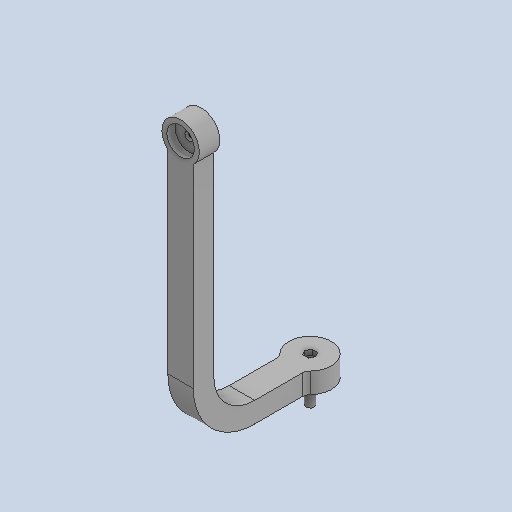
# Autodesk Inventor part: distal_link_2
Saved by Autodesk Inventor 2024 (Build 280153000, 153)
## iProperties
Created: 2023-10-30
Part Number: distal_link_2
Material: Generic
Document SubType Name: Modeling
Designer: MATEO
Density: 1 g/cm^3
Appearance: Default
Author: MATEO
Autodesk Inventor part; units mm, degrees
ref_plane "YZ Plane" through (0, 0, 0) normal (1, 0, 0) x (0, 1, 0)
ref_plane "XZ Plane" through (0, 0, 0) normal (0, 1, 0) x (-1, 0, 0)
sketch "Sketch1" plane through (0, 0, 0) normal (0, 1, 0) x (-1, 0, 0)
  arc A0 (-8.9286, 8.7482) -> (8.9286, 8.7482) centre (0, 0) ccw
  line L0 (-7.5, 12.2474) -> (-7.5, 20)
  line L1 (7.5, 20) -> (7.5, 12.2474)
  line L2 (7.5, 20) -> (-7.5, 20)
  arc A1 (7.5, 12.2474) -> (8.9286, 8.7482) centre (12.5, 12.2474) ccw
  arc A2 (-8.9286, 8.7482) -> (-7.5, 12.2474) centre (-12.5, 12.2474) ccw
  point P0 (7.5, 10)
  point P1 (-7.5, 10)
  point P2 (0, 10)
  point P3 (0, 20)
  dimension "d0" = 25
  dimension "d109" = 5
  dimension "d129" = 15
  dimension "d131" = 10
  constraints: 8 point on circle, 6 end point, 5 horizontal alignment, 4 tangent, 3 centre point, 2 point on line, 2 vertical alignment, 1 coincident, 1 equal radius, 1 midpoint, 1 parallel
  measures "d0" diameter of A0
  measures "d109" radius of A1
  measures "d129" distance of L1.start L0.end
  measures "d131" distance from line of L2 point (0, 10)
extrude "Extrusion1" add sketch "Sketch1" against normal blind 12
sketch "Sketch22" plane through (-7.5, 0, 20) normal (0, 0, 1) x (1, 0, 0)
  line L0 (0, 0) -> (0, -12) projected
  line L1 (15, -12) -> (0, -12) projected
  line L2 (0, 0) -> (15, 0)
  line L3 (15, 0) -> (15, -12)
  line L4 (15, -12) -> (0, -12)
  line L5 (0, -12) -> (0, 0)
  point P0 (7.5, 0)
  constraints: 8 end point, 2 parallel, 1 horizontal, 1 perpendicular
sketch "Sketch23" plane through (0, 0, 0) normal (1, 0, 0) x (0, 1, 0)
  line L0 (0, 20) -> (-12, 20) projected
  line L1 (-6, 20) -> (-6, 40)
  line L2 (24, 70) -> (134.0108, 70)
  arc A0 (24, 70) -> (-6, 40) centre (24, 40) ccw
  point P0 (0, 0)
  point P1 (-6, 70)
  dimension "d110" = 50
  dimension "d111" = 140.0108
  dimension "d112" = 90
  dimension "d113" = 30
  constraints: 4 end point, 2 point on circle, 2 point on line, 2 tangent, 1 centre point, 1 midpoint, 1 vertical
  measures "d110" distance of L1.start point (-6, 70)
  measures "d111" distance of point (-6, 70) L2.end
  measures "d112" angle of L1 L2
  measures "d113" radius of A0
sweep "Sweep2" add profiles "Sketch22" path "Sketch23" path curves L1 A0 L2
ref_plane "Work Plane11" through (7.5, 24, 70) normal (0, 0, -1) x (-1, 0, 0)
sketch "Sketch24" plane through (7.5, 24, 70) normal (0, 0, -1) x (-1, 0, 0)
  line L0 (0, 110.0108) -> (15, 110.0108)
  line L1 (0, 110.0108) -> (15, 110.0108)
  line L2 (0, 110.0108) -> (0, 113.964)
  line L3 (15, 110.0108) -> (15, 113.964)
  arc A0 (15, 113.964) -> (0, 113.964) centre (7.5, 122.0108) ccw
  line L4 (0, 110.0108) -> (15, 110.0108) projected
  point P0 (7.5, -24)
  point P1 (7.5, 110.0108)
  point P2 (7.5, 110.0108)
  dimension "d139" = 22
  dimension "d140" = 12
  dimension "d141" = 15
  constraints: 8 end point, 4 horizontal alignment, 3 midpoint, 2 coincident, 2 point on circle, 2 vertical, 1 centre point, 1 collinear, 1 vertical alignment
  measures "d139" diameter of A0
  measures "d140" distance from line of L0 A0.centre
  measures "d141" distance of L0.start L0.end
extrude "Extrusion17" add sketch "Sketch24" along normal mid plane 12
sketch "Sketch25" plane through (-7.5, 24, 76) normal (0, 0, 1) x (1, 0, 0)
  circle A0 centre (7.5, 122.0108) radius 2.5
  arc A1 (15, 113.964) -> (0, 113.964) centre (7.5, 122.0108) ccw projected
  point P0 (7.5, -24)
  dimension "d123" = 5
  constraints: 2 coincident, 1 centre point
  measures "d123" diameter of A0
extrude "Extrusion18" cut sketch "Sketch25" against normal through all
sketch "Sketch27" plane through (0, 0, 0) normal (0, 1, 0) x (1, 0, 0)
  arc A0 (8.9286, -8.7482) -> (-8.9286, -8.7482) centre (0, 0) ccw projected
  circle A1 centre (0, 0) radius 2.4
  dimension "d136" = 4.8
  constraints: 1 centre point, 1 coincident
  measures "d136" diameter of A1
extrude "Extrusion20" add sketch "Sketch27" against normal blind 26
sketch "Sketch28" plane through (7.5, 24, 64) normal (0, 0, -1) x (-1, 0, 0)
  circle A0 centre (7.5, 122.0108) radius 2.5 projected
  circle A1 centre (7.5, 122.0108) radius 8.1
  point P0 (7.5, -24)
  dimension "d142" = 16.2
  constraints: 1 centre point, 1 coincident
  measures "d142" diameter of A1
extrude "Extrusion21" cut sketch "Sketch28" against normal blind 5
mirror "Mirror2" about plane through (7.5, 24, 70) normal (0, 0, -1) of "Extrusion21"
sketch "Sketch29" plane through (0, 0, 0) normal (0, 1, 0) x (1, 0, 0)
  circle A0 centre (0, 0) radius 2.4 projected
  line L0 (3.1754, 0) -> (1.5877, -2.75)
  line L1 (1.5877, -2.75) -> (-1.5877, -2.75)
  line L2 (-1.5877, -2.75) -> (-3.1754, 0)
  line L3 (-3.1754, 0) -> (-1.5877, 2.75)
  line L4 (-1.5877, 2.75) -> (1.5877, 2.75)
  line L5 (1.5877, 2.75) -> (3.1754, 0)
  dimension "d145" = 5.5
  constraints: 12 end point, 1 coincident, 1 horizontal alignment, 13 other
  measures "d145" distance between parallel lines of L1 L4
extrude "Extrusion22" cut sketch "Sketch29" against normal blind 3 contours A0 | L0 L1 L2 L3 L4 L5
sketch "Sketch30" plane through (0, -3, 0) normal (0, 1, 0) x (1, 0, 0)
  circle A0 centre (0, 0) radius 1.6
  dimension "d148" = 3.2
  constraints: 1 centre point, 1 coincident
  measures "d148" diameter of A0
extrude "Extrusion23" cut sketch "Sketch30" against normal through all
body "Solid1"
